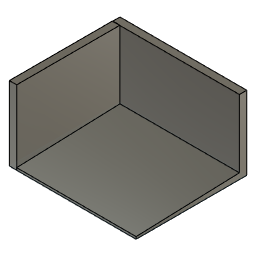
ScoopWIP v1 (Autodesk Fusion 360 design; units mm, degrees)
Autodesk Fusion 360 part; units mm, degrees
sketch "Sketch1" plane through (0, 0, 0) normal (0, 0, 1) x (1, 0, 0)
  line L0 (0, 90) -> (81, 90)
  line L1 (81, 90) -> (81, 19.9574)
  line L2 (81, 19.9574) -> (0, 19.9574)
  line L3 (0, 19.9574) -> (0, 90)
  dimension "d1" = 81
  constraint horizontal L0
  constraint vertical L1
  constraint horizontal L2
  constraint vertical L3
  measures "d1" distance of L0.start L0.end
extrude "Extrude1" add sketch "Sketch1" along normal blind 4
draft "Draft1" angle -2 neutral plane through (0, 90, 0) pull (0, 1, 0) 1 faces at (27, 66.6525, 4)
sketch "Sketch2" plane through (0, 0, 0) normal (1, 0, 0) x (0, 1, 0)
  line L0 (20, 0) -> (90, 0)
  line L1 (90, 0) -> (90, 50.1733)
  line L2 (90, 50.1733) -> (20, 50.1733)
  line L3 (20, 50.1733) -> (20, 0)
  dimension "d6" = 70
  constraint horizontal L0
  constraint vertical L1
  constraint horizontal L2
  constraint vertical L3
  measures "d6" distance of L0.start L0.end
extrude "Extrude2" add sketch "Sketch2" against normal blind 5
sketch "Sketch3" plane through (0, 0, 0) normal (0, 1, 0) x (1, 0, 0)
  line L0 (-5, 0, 90) -> (81, 0, 90)
  line L1 (81, 0, 90) -> (81, -50, 90)
  line L2 (81, -50, 90) -> (-5, -50, 90)
  line L3 (-5, -50, 90) -> (-5, 0, 90)
extrude "Extrude3" add sketch "Sketch3" along normal blind 5 contours L0 L1 L2 L3 in plane through (0, 90, 0) normal (0, 1, 0)
sketch "Sketch4" plane through (0, 0, 0) normal (0, 0, -1) x (1, 0, 0)
  line L0 (81, -19.9574) -> (0, -19.9574)
  line L1 (0, -19.9574) -> (0, -20)
  line L2 (0, -20) -> (-5, -20)
  line L3 (-5, -20) -> (-5, -95)
  line L4 (-5, -95) -> (81, -95)
  line L5 (81, -95) -> (81, -19.9574)
sketch "Sketch5" plane through (0, 0, 0) normal (0, 0, 1) x (1, 0, 0)
sketch "Sketch6" plane through (0, 0, 0) normal (1, 0, 0) x (0, 1, 0)
sketch "Sketch7" plane through (0, 0, 0) normal (1, 0, 0) x (0, 1, 0)
